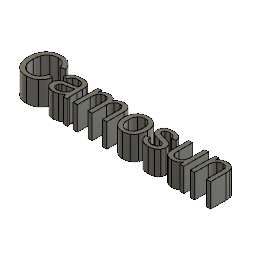
_CamosunText.939b9878-5a56-477e-b37d-910154077e00 (Autodesk Fusion 360 design; units mm, degrees)
Autodesk Fusion 360 part; units mm, degrees
form "Form1" [no effect]
sketch "Sketch1" plane through (0, 0, 0) normal (0, 1, 0) x (1, 0, 0)
  line L0 (5.0007, -8.3147) -> (46.612, -8.3147) construction
  line L1 (46.612, -8.3147) -> (46.612, 1.6853) construction
  line L2 (46.612, 1.6853) -> (5.0007, 1.6853) construction
  line L3 (5.0007, 1.6853) -> (5.0007, -8.3147) construction
  text T0 "Camosun" font "Arial" height 10 align ink ink in box 0 x 0 at (5.0007, -8.3147) x (1, 0) y (0, 1) spacing 1 height is em
extrude "Extrude1" add sketch "Sketch1" along normal blind 5 and the other way blind 0 text T0 makes body 1 at (16.2914, 0, 6.7054) makes body 2 at (42.4081, 1.6667, 6.449) makes body 3 at (25.9832, 2.5, 5.1503) makes body 4 at (41.0312, 1.6667, 4.7204) makes body 5 at (34.2408, 0, 5.5058) makes body 6 at (17.955, 1.6667, 6.449) makes body 7 at (5.3682, 0, 4.1159)
